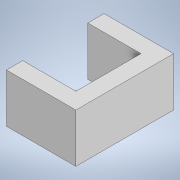
# Autodesk Inventor part: MotorMountTest
Saved by Autodesk Inventor 2021 (Build 250183000, 183)
## iProperties
Created: 2021-09-12
Part Number: MotorMountTest
Material: Generic
Document SubType Name: Modeling
Designer: ermoz
Density: 1 g/cm^3
Appearance: Default
Author: ermoz
Autodesk Inventor part; units mm, degrees
ref_plane "YZ Plane" through (0, 0, 0) normal (1, 0, 0) x (0, 1, 0)
ref_plane "XZ Plane" through (0, 0, 0) normal (0, 1, 0) x (-1, 0, 0)
ref_plane "XY Plane" through (0, 0, 0) normal (0, 0, 1) x (1, 0, 0)
sketch "Sketch1" plane through (0, 0, 0) normal (0, 1, 0) x (-1, 0, 0)
  line L0 (-3.364, -7.7022) -> (6.436, -7.7022)
  line L1 (6.436, -7.7022) -> (6.436, 4.2978)
  line L2 (6.436, 4.2978) -> (-3.364, 4.2978)
  line L3 (-3.364, 4.2978) -> (-3.364, -7.7022)
  line L4 (-3.364, -7.7022) -> (6.436, 4.2978) construction
  line L5 (6.436, -7.7022) -> (-3.364, 4.2978) construction
  line L6 (6.436, 4.2978) -> (6.436, 7.2978)
  line L7 (6.436, 7.2978) -> (-6.364, 7.2978)
  line L8 (-6.364, 7.2978) -> (-6.364, -10.7022)
  line L9 (-6.364, -10.7022) -> (6.436, -10.7022)
  line L10 (6.436, -10.7022) -> (6.436, -7.7022)
  point P0 (1.536, -1.7022)
  dimension "d27" = 12
  dimension "d28" = 9.8
  dimension "d29" = 3
  dimension "d30" = 3
  constraints: 22 end point, 5 perpendicular, 2 midpoint, 2 parallel, 2 point on line, 1 collinear, 1 horizontal
  measures "d27" distance of L0.end L1.end
  measures "d28" distance of L1.end L2.end
  measures "d29" distance of L1.end L6.end
  measures "d30" distance between parallel lines of L8 L3
extrude "Extrusion1" add sketch "Sketch1" along normal blind 9 contours L0 L10 L9 L8 L7 L6 L2 L3
sketch "Sketch2" plane through (0, 9, 0) normal (0, 1, 0) x (1, 0, 0)
  line L0 (3.364, -0.7978) -> (2.864, -0.7978)
  line L1 (2.864, -0.7978) -> (2.864, -2.2978)
  line L2 (-0.136, -4.2978) -> (-0.136, -3.7978)
  line L3 (-0.136, -4.2978) -> (0.364, -4.2978) construction
  line L4 (-0.136, -3.7978) -> (1.364, -3.7978)
  arc A0 (1.364, -3.7978) -> (2.864, -2.2978) centre (1.364, -2.2978) ccw
  line L5 (-0.136, -4.2978) -> (3.364, -4.2978)
  line L6 (3.364, -4.2978) -> (3.364, -0.7978)
  line L7 (3.364, 7.7022) -> (3.364, -4.2978) projected
  line L8 (3.364, -4.2978) -> (-6.436, -4.2978) projected
  point P0 (0, 0)
  point P1 (5, 6)
  point P2 (5, -6.1)
  dimension "d8" = 0.5
  dimension "d9" = 0.5
  dimension "d10" = 90
  dimension "d13" = 1.5
  dimension "d31" = 3.5
  dimension "d32" = 3.5
  constraints: 15 end point, 4 perpendicular, 3 horizontal, 2 collinear, 2 point on circle, 2 tangent, 1 centre point, 1 vertical
  measures "d8" distance of L0.start L0.end
  measures "d9" distance of L2.start L2.end
  measures "d10" angle of L3 L2
  measures "d13" radius of A0
  measures "d31" distance of L5.end L0.start
  measures "d32" distance of L2.start L5.end
extrude "Extrusion2" add sketch "Sketch2" against normal up to surface (9 mm away)
sketch "Sketch3" plane through (-0.136, 9, 3.7978) normal (-1, 0, 0) x (0, 0, 1)
  line L0 (0.5, 0) -> (3.5, 0) projected
  line L1 (0.5, 0) -> (-3, 0)
  line L2 (-3, 0) -> (-3, -0.875)
  line L3 (-3, -0.875) -> (0.5, -0.875)
  line L4 (0.5, -0.875) -> (0.5, 0)
  line L5 (-3, 0) -> (-3, -9) projected
  line L6 (0.5, 0) -> (0.5, -9) projected
  line L7 (-3, -9) -> (-3, 0) projected
  line L8 (0.5, -9) -> (-3, -9)
  line L9 (-3, -9) -> (-3, -8.125)
  line L10 (-3, -8.125) -> (0.5, -8.125)
  line L11 (0.5, -8.125) -> (0.5, -9)
  line L12 (0.5, -5.875) -> (-3, -5.875)
  line L13 (-3, -5.875) -> (-3, -4.875)
  line L14 (-3, -4.875) -> (0.5, -4.875)
  line L15 (0.5, -4.875) -> (0.5, -5.875)
  point P0 (0.5, -8.125)
  point P1 (0.5, -4.875)
  dimension "d33" = 0.875
  dimension "d34" = 0.875
  dimension "d35" = 4
  dimension "d36" = 1
  constraints: 24 end point, 6 parallel, 3 horizontal, 3 perpendicular, 3 point on line, 1 collinear
  measures "d33" distance of L2.end L1.end
  measures "d34" distance between parallel lines of L10 L8
  measures "d35" distance between parallel lines of L3 L14
  measures "d36" distance of L12.end L13.end
extrude "Extrusion3" cut sketch "Sketch3" against normal up to surface (3.5 mm away) contours L4 L3 L2 L1 | L6 L12 L5 L14 | L6 L8 L5 L10
body "Solid1"
